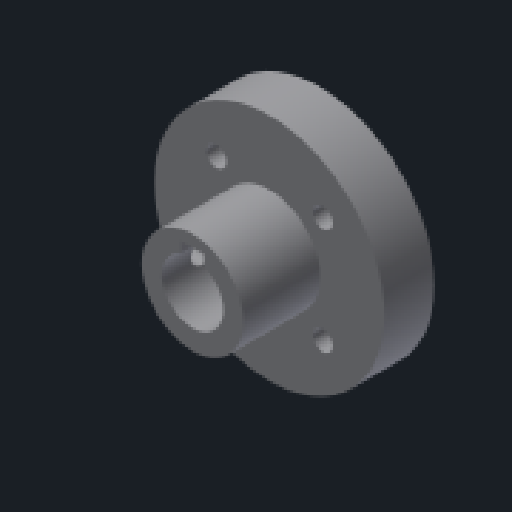
# Autodesk Inventor part: BaseHub
Saved by Autodesk Inventor 2023 (Build 270158000, 158)
## iProperties
Created: 2024-01-25
Part Number: BaseHub
Material: Generic
Document SubType Name: Modeling
Designer: valer
Density: 1 g/cm^3
Appearance: Default
Author: valer
Autodesk Inventor part; units mm, degrees
ref_plane "YZ Plane" through (0, 0, 0) normal (1, 0, 0) x (0, 1, 0)
ref_plane "XZ Plane" through (0, 0, 0) normal (0, 1, 0) x (-1, 0, 0)
ref_plane "XY Plane" through (0, 0, 0) normal (0, 0, 1) x (1, 0, 0)
sketch "Sketch1" plane through (0, 0, 0) normal (0, 0, 1) x (1, 0, 0)
  circle A0 centre (0, 0) radius 6.6 construction
  circle A1 centre (-6.9148, 6.9148) radius 1.5875 construction
  circle A2 centre (6.9148, 6.9148) radius 1.5875 construction
  circle A3 centre (-6.9148, -6.9148) radius 1.5875 construction
  circle A4 centre (6.9148, -6.9148) radius 1.5875 construction
  line L0 (-6.9148, 6.9148) -> (6.9148, 6.9148) construction
  line L1 (6.9148, 6.9148) -> (6.9148, -6.9148) construction
  line L2 (6.9148, -6.9148) -> (-6.9148, -6.9148) construction
  line L3 (-6.9148, -6.9148) -> (-6.9148, 6.9148) construction
  circle A5 centre (0, 0) radius 12.958 construction
  line L4 (-6.9148, -6.9148) -> (6.9148, 6.9148) construction
  line L5 (-6.9148, 6.9148) -> (-5.7923, 5.7923) construction
  line L6 (-5.7923, 5.7923) -> (-4.6669, 4.6669) construction
  line L7 (-8.0373, 8.0373) -> (-9.1627, 9.1627) construction
  circle A6 centre (0, 0) radius 4
  line L8 (0, 4) -> (0, 5.05) construction
  line L9 (0, -20.9412) -> (0, 20.9412) construction
  line L10 (-1.475, 5.05) -> (1.475, 5.05)
  line L11 (-1.475, 5.05) -> (-1.475, 3.7181)
  line L12 (1.475, 5.05) -> (1.475, 3.7181)
  circle A7 centre (0, 0) radius 14.958
  circle A8 centre (6.9148, 6.9148) radius 1.2891
  circle A9 centre (6.9148, -6.9148) radius 1.2891
  circle A10 centre (-6.9148, -6.9148) radius 1.2891
  circle A11 centre (-6.9148, 6.9148) radius 1.2891
  dimension "d0" = 13.2
  dimension "d1" = 3.175
  dimension "d5" = 13.8296
  dimension "d6" = 45
  dimension "d9" = 8
  dimension "d10" = 1.05
  dimension "d11" = 2.95
  dimension "d14" = 2
  dimension "d15" = 29.916
  dimension "d21" = 2.5781
  constraints: 24 end point, 13 coincident, 10 centre point, 6 equal radius, 5 point on circle, 3 collinear, 3 vertical, 2 equal length, 2 horizontal, 2 midpoint, 2 parallel, 1 perpendicular, 6 other
  measures "d1" diameter of A1
  measures "d5" distance of L0.start L0.end
  measures "d6" angle of L0 L5
  measures "d9" diameter of A6
  measures "d10" distance of L8.end L8.start
  measures "d11" distance of L10.start L10.end
  measures "d15" diameter of A7
  measures "d21" diameter of A8
extrude "HubFeature" add sketch "Sketch1" against normal blind 6.5
sketch "Sketch2" plane through (0, 0, 0) normal (0, 0, 1) x (1, 0, 0)
  circle A0 centre (0, 0) radius 6.6 projected
  line L0 (-1.475, 5.05) -> (1.475, 5.05) projected
  line L1 (-1.475, 3.7181) -> (-1.475, 5.05) projected
  line L2 (1.475, 5.05) -> (1.475, 3.7181) projected
  arc A1 (-1.475, 3.7181) -> (1.475, 3.7181) centre (0, 0) ccw projected
extrude "LipFeature" add sketch "Sketch2" along normal blind 10
sketch "Sketch3" plane through (0, 0, -6.5) normal (0, 0, -1) x (-1, 0, 0)
  circle A0 centre (0, 0) radius 12
  dimension "d18" = 24
  constraints: 1 centre point, 1 coincident
  measures "d18" diameter of A0
extrude "BearingIndentFeature" cut sketch "Sketch3" against normal blind 3.5
sketch "SetScrewHole" plane through (0, 0, 0) normal (1, 0, 0) x (0, 1, 0)
  line L0 (6.6, 10) -> (-6.6, 10) construction
  line L1 (-6.6, 0) -> (6.6, 0) construction
  line L2 (-4, 10) -> (3.7181, 10) construction
  circle A0 centre (0, 6.5) radius 1.25
  line L3 (0, 10) -> (0, 0) construction
  line L4 (14.958, 0) -> (-14.958, 0) projected
  dimension "d22" = 2.5
  dimension "d25" = 3.5
  constraints: 2 end point, 2 point on line, 1 centre point, 1 coincident, 1 perpendicular
  measures "d22" diameter of A0
  measures "d25" distance from line of L0 A0.centre
extrude "SetScrewHoleFeature" cut sketch "SetScrewHole" against normal through all
body "Solid1"
